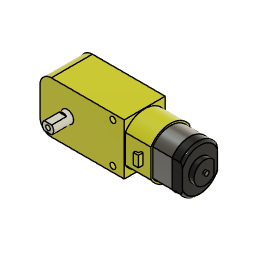
TT_MOTOR_DUAL_AXLE v4 (Autodesk Fusion 360 design; units mm, degrees)
Autodesk Fusion 360 part; units mm, degrees
note: some values were not read from the file. Set by a fixed rule: which face or edge a step refers to.
sketch "YellowBodyMain" plane through (0, 0, 0) normal (0, 0, 1) x (1, 0, 0)
  line L0 (-12, 9) -> (25, 9)
  line L1 (25, 9) -> (25, -9)
  line L2 (25, -9) -> (-12, -9)
  line L3 (-12, -9) -> (-12, 9)
  point P0 (-12, 0)
  dimension "d1" = 37
  dimension "d2" = 18
  dimension "d3" = 12
  constraint horizontal L0
  constraint vertical L1
  constraint horizontal L2
  constraint vertical L3
  constraint midpoint L3 P0
  constraint horizontal origin P0
  measures "d1" distance of L0.start L0.end
  measures "d2" distance of L0.start L2.end
  measures "d3" distance of origin L3
extrude "Extrude1" add sketch "YellowBodyMain" along normal mid plane 22.5 makes body 1
fillet "Fillet1" radius 5 2 edges at (-12, 0, -11.25) (-12, 0, 11.25) on bodies 1
sketch "YellowFrontTab" plane through (-12, 0, 0) normal (-1, 0, 0) x (0, -1, 0)
  line L0 (9, 6.25) -> (-9, 6.25)
  line L1 (-9, 6.25) -> (-9, -6.25)
  line L2 (-9, -6.25) -> (9, -6.25)
  line L3 (9, -6.25) -> (9, 6.25)
  line L4 (-1.5, 2.5) -> (1.5, 2.5)
  line L5 (1.5, 2.5) -> (1.5, -2.5)
  line L6 (1.5, -2.5) -> (-1.5, -2.5)
  line L7 (-1.5, -2.5) -> (-1.5, 2.5)
  line L8 (-1.5, 2.5) -> (1.5, -2.5) construction
  line L9 (1.5, 2.5) -> (-1.5, -2.5) construction
  dimension "d8" = 3
  dimension "d9" = 5
  constraint horizontal L4
  constraint perpendicular L4 L5
  constraint parallel L4 L6
  constraint parallel L5 L7
  constraint coincident L8 origin
  constraint coincident L9 origin
  measures "d8" distance of L5.end L6.end
  measures "d9" distance of L4.end L5.end
extrude "Extrude2" add sketch "YellowFrontTab" along normal blind 5 contours L4 L5 L6 L7 bodies 1
sketch "YellowFrontTabHole" plane through (0, -1.5, 0) normal (0, -1, 0) x (1, 0, 0)
  line L0 (-12, -2.5) -> (-12, 2.5)
  line L1 (-12, 2.5) -> (-17, 2.5)
  line L2 (-17, 2.5) -> (-17, -2.5)
  line L3 (-17, -2.5) -> (-12, -2.5)
  circle A0 centre (-14.5, 0) radius 1.25
  point P0 (-17, 0)
  point P1 (-14.5, 2.5)
  dimension "d12" = 2.5
  constraint midpoint L2 P0
  constraint horizontal A0.centre P0
  constraint midpoint L1 P1
  constraint vertical A0.centre P1
  measures "d12" diameter of A0
extrude "Extrude3" cut sketch "YellowFrontTabHole" against normal blind 3 contours A0 bodies 1
sketch "Yellow Body holes" plane through (0, 9, 0) normal (0, 1, 0) x (-1, 0, 0)
  arc A0 (12, 6.25) -> (7, 11.25) centre (7, 6.25) ccw
  line L0 (7, 11.25) -> (-25, 11.25)
  line L1 (-25, 11.25) -> (-25, -11.25)
  line L2 (-25, -11.25) -> (7, -11.25)
  arc A1 (7, -11.25) -> (12, -6.25) centre (7, -6.25) ccw
  line L3 (12, -6.25) -> (12, 6.25)
  circle A2 centre (-20, -8.75) radius 1.25
  line L4 (-1.75, 0) -> (-22.5, 0)
  circle A3 centre (-20, 8.75) radius 1.25
  dimension "d15" = 2.5
  dimension "d16" = 5
  dimension "d17" = 2.5
  constraint symmetric A2 L4 A3
  measures "d15" diameter of A2
  measures "d16" distance of L1 A2.centre
  measures "d17" distance of L2 A2.centre
extrude "Extrude4" cut sketch "Yellow Body holes" against normal up to surface (18 mm away) contours A2 | A3 bodies 1
sketch "YellowBodyBoss" plane through (0, 9, 0) normal (0, 1, 0) x (-1, 0, 0)
  circle A0 centre (-20, -8.75) radius 1.25
  circle A1 centre (-20, 8.75) radius 1.25
  arc A2 (12, 6.25) -> (7, 11.25) centre (7, 6.25) ccw
  line L0 (7, 11.25) -> (-25, 11.25)
  line L1 (-25, 11.25) -> (-25, -11.25)
  line L2 (-25, -11.25) -> (7, -11.25)
  arc A3 (7, -11.25) -> (12, -6.25) centre (7, -6.25) ccw
  line L3 (12, -6.25) -> (12, 6.25)
  circle A4 centre (-11, 0) radius 2
  dimension "d20" = 4
  dimension "d21" = 14
  constraint horizontal origin A4.centre
  measures "d20" diameter of A4
  measures "d21" distance of L1 A4.centre
extrude "Extrude5" add sketch "YellowBodyBoss" along normal blind 1.5 contours A4 bodies 1
sketch "YellowMotorHousing" plane through (25, 0, 0) normal (1, 0, 0) x (0, 1, 0)
  line L0 (9, -11.25) -> (9, 11.25)
  line L1 (9, 11.25) -> (-9, 11.25)
  line L2 (-9, 11.25) -> (-9, -11.25)
  line L3 (-9, -11.25) -> (9, -11.25)
  line L4 (8.5, -6.25) -> (8.5, 6.25)
  line L5 (-8.5, -6.25) -> (-8.5, 6.25)
  line L6 (8.5, -6.25) -> (-8.5, -6.25) construction
  line L7 (0, -11) -> (0, 11) construction
  arc A0 (-8.5, -6.25) -> (8.5, -6.25) centre (0, -1.0197) ccw
  arc A1 (8.5, 6.25) -> (-8.5, 6.25) centre (0, 1.0197) ccw
  point P0 (8.5, -6.25)
  point P1 (-8.5, -6.25)
  point P2 (8.5, 6.25)
  point P3 (-8.5, 6.25)
  point P4 (8.5, 0)
  point P5 (0, -6.25)
  point P6 (0, -11)
  point P7 (0, 11)
  dimension "d24" = 17
  dimension "d25" = 12.5
  dimension "d26" = 22
  constraint horizontal P0 P1
  constraint horizontal P2 P3
  constraint vertical P0 P2
  constraint vertical P1 P3
  constraint coincident P0 L4.start
  constraint coincident P2 L4.end
  constraint coincident P1 L5.start
  constraint coincident P3 L5.end
  constraint midpoint L4 P4
  constraint horizontal origin P4
  constraint midpoint L6 P5
  constraint vertical origin P5
  constraint coincident P6 L7.start
  constraint coincident P7 L7.end
  constraint perpendicular L1 L7
  constraint midpoint L7 origin
  constraint coincident P6 A0
  constraint coincident P7 A1
  measures "d24" distance of P0 P1
  measures "d25" distance of P1 P3
  measures "d26" distance of P6 P7
extrude "Extrude6" add sketch "YellowMotorHousing" along normal blind 11.25 thin wall 0.8 inside contours L4 L5 A0 A1 bodies 1
sketch "YellowBodyHook" plane through (0, 8.5, 0) normal (0, 1, 0) x (-1, 0, 0)
  line L0 (-25, -6.25) -> (-25, 6.25)
  line L1 (-25, 6.25) -> (-36.25, 6.25)
  line L2 (-36.25, 6.25) -> (-36.25, -6.25)
  line L3 (-36.25, -6.25) -> (-25, -6.25)
  line L4 (-31.75, -2.375) -> (-32.75, -2.375)
  line L5 (-32.75, -2.375) -> (-32.75, 2.375)
  line L6 (-32.75, 2.375) -> (-31.75, 2.375)
  line L7 (-31.75, 2.375) -> (-31.75, -2.375)
  line L8 (-31.75, -2.375) -> (-32.75, 2.375) construction
  line L9 (-32.75, -2.375) -> (-31.75, 2.375) construction
  point P0 (-32.25, 0)
  dimension "d30" = 1
  dimension "d31" = 4.75
  dimension "d32" = 3.5
  constraint horizontal L4
  constraint perpendicular L4 L5
  constraint parallel L4 L6
  constraint parallel L5 L7
  constraint coincident L8 P0
  constraint coincident L9 P0
  measures "d30" distance of L5.end L6.end
  measures "d31" distance of L4.end L5.end
  measures "d32" distance of L2 L5
extrude "Extrude7" add sketch "YellowBodyHook" along normal blind 2 contours L4 L5 L6 L7 bodies 1
sketch "YellowBodyHookSides" plane through (32.75, 0, 0) normal (1, 0, 0) x (0, 1, 0)
  line L0 (8.5, 2.375) -> (8.5, -2.375)
  line L1 (8.5, -2.375) -> (10.5, -2.375)
  line L2 (10.5, -2.375) -> (10.5, 2.375)
  line L3 (10.5, 2.375) -> (8.5, 2.375)
  line L4 (10.5, -2.375) -> (9.5, -2.375)
  line L5 (9.5, -2.375) -> (9.5, 2.375)
  line L6 (9.5, 2.375) -> (10.5, 2.375)
  line L7 (10.5, 2.375) -> (10.5, -2.375)
  dimension "d35" = 1
  constraint horizontal L4
  constraint vertical L5
  constraint horizontal L6
  constraint vertical L7
  constraint coincident L1.end L2.start
  constraint collinear L3 L6
  measures "d35" distance of L1.end L4.end
extrude "Extrude8" add sketch "YellowBodyHookSides" against normal blind 2.25 contours L1 L2 L3 L4 L5 L6 L7 bodies 1
mirror "Mirror1" about plane through (0, 0, 0) normal (0, 1, 0) of "Extrude7", "Extrude8"
sketch "YellowShaftHole" plane through (0, 9, 0) normal (0, 1, 0) x (-1, 0, 0)
  circle A0 centre (-11, 0) radius 2
  circle A1 centre (-20, -8.75) radius 1.25
  circle A2 centre (-20, 8.75) radius 1.25
  arc A3 (12, 6.25) -> (7, 11.25) centre (7, 6.25) ccw
  line L0 (7, 11.25) -> (-25, 11.25)
  line L1 (-25, 11.25) -> (-25, -11.25)
  line L2 (-25, -11.25) -> (7, -11.25)
  arc A4 (7, -11.25) -> (12, -6.25) centre (7, -6.25) ccw
  line L3 (12, -6.25) -> (12, 6.25)
  circle A5 centre (0, 0) radius 2.75
  dimension "d54" = 5.5
  constraint coincident A5.centre origin
  measures "d54" diameter of A5
extrude "Extrude13" cut sketch "YellowShaftHole" against normal up to surface (18 mm away) contours A5 bodies 1
extrude "Extrude9" add 1 faces at (25, -2.5667, 2.0062) along direction (1, 0, 0) blind 8.5 from surface at 11.25 separate body on bodies 1 makes body 2
extrude "Extrude10" add 1 faces at (44.75, -2.5667, 2.0062) along direction (1, 0, 0) blind 4.5 separate body on bodies 2 makes body 3
fillet "Fillet2" radius 1 2 edges at (49.25, 0, -10.2) (49.25, 0, 10.2) on bodies 3
sketch "MotorBlackCircle" plane through (49.25, 0, 0) normal (1, 0, 0) x (0, 1, 0)
  arc A0 (7.7, 3.7814) -> (-7.7, 3.7814) centre (0, 1.0197) ccw
  line L0 (-7.7, 3.7814) -> (-7.7, -3.7814)
  arc A1 (-7.7, -3.7814) -> (7.7, -3.7814) centre (0, -1.0197) ccw
  line L1 (7.7, -3.7814) -> (7.7, 3.7814)
  circle A2 centre (0, 0) radius 4.875
  line L2 (3.925, 2.8914) -> (3.925, -2.8914)
  line L3 (3.925, 0) -> (-4.875, 0) construction
  dimension "d47" = 9.75
  dimension "d48" = 8.8
  constraint coincident A2.centre origin
  constraint coincident A2 L2.start
  constraint coincident A2 L2.end
  constraint vertical L2
  constraint midpoint L2 L3.start
  constraint coincident A2 L3.end
  constraint perpendicular L2 L3
  measures "d47" diameter of A2
  measures "d48" distance of L3.start L3.end
extrude "Extrude11" add sketch "MotorBlackCircle" along normal blind 2.26 contours A2 L2 picked at (0.3361, -0.2387) bodies 3
sketch "MotorMetalShaft" plane through (51.51, 0, 0) normal (1, 0, 0) x (0, 1, 0)
  arc A0 (3.925, 2.8914) -> (3.925, -2.8914) centre (0, 0) ccw
  line L0 (3.925, -2.8914) -> (3.925, 2.8914)
  circle A1 centre (0, 0) radius 0.95
  dimension "d51" = 1.9
  constraint coincident A0.centre A1.centre
  measures "d51" diameter of A1
extrude "Extrude12" add sketch "MotorMetalShaft" along normal blind 0.8 separate body contours A1 makes body 4
sketch "DriveAxle" plane through (0, 0, 0) normal (0, 1, 0) x (1, 0, 0)
  circle A0 centre (0, 0) radius 2.5
  dimension "d58" = 5
  constraint coincident A0.centre origin
  measures "d58" diameter of A0
extrude "Extrude14" add sketch "DriveAxle" along normal mid plane 22 separate body makes body 5
sketch "DriveAxleFlat" plane through (0, -11, 0) normal (0, -1, 0) x (1, 0, 0)
  circle A0 centre (0, 0) radius 2.5
  line L0 (-1.6536, 1.875) -> (1.6536, 1.875)
  line L1 (-1.6536, -1.875) -> (1.6536, -1.875)
  circle A1 centre (0, 0) radius 1
  dimension "d61" = 3.75
  dimension "d62" = 2
  constraint coincident A0 L0.start
  constraint coincident A0 L0.end
  constraint horizontal L0
  constraint coincident A0 L1.start
  constraint coincident A0 L1.end
  constraint parallel L0 L1
  constraint vertical L0.start L1.start
  constraint concentric A0 A1
  measures "d61" distance of L0 L1
  measures "d62" diameter of A1
extrude "Extrude15" add sketch "DriveAxleFlat" along normal blind 6.5 contours A0 L0 L1 bodies 5
extrude "Extrude16" add sketch "DriveAxleFlat" against normal blind 6.5 from surface at -22 contours A0 L0 L1 bodies 5
named bodies: "YellowBody", "MotorMetal"
